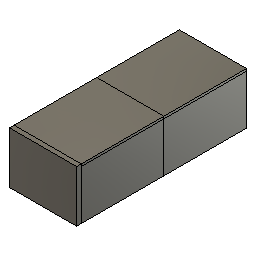
return_to_box_split (Autodesk Fusion 360 design; units mm, degrees)
Autodesk Fusion 360 part; units mm, degrees
sketch "Sketch1" plane through (0, 0, 0) normal (0, 0, 1) x (1, 0, 0)
  line L0 (0, 0) -> (117, 0)
  line L1 (117, 0) -> (117, 86)
  line L2 (117, 86) -> (0, 86)
  line L3 (0, 86) -> (0, 0)
  dimension "d1" = 86
  dimension "d2" = 117
  constraint horizontal L0
  constraint vertical L1
  constraint horizontal L2
  constraint vertical L3
  constraint coincident L0.start L3.end
  measures "d1" distance of L0.end L1.end
  measures "d2" distance of L0.start L0.end
extrude "Extrude1" add sketch "Sketch1" along normal blind 5 makes body 1
sketch "Sketch2" plane through (0, 0, 5) normal (0, 0, 1) x (1, 0, 0)
  line L0 (0, 86) -> (0, 0)
  line L1 (0, 0) -> (117, 0)
  line L2 (117, 0) -> (117, 86)
  line L3 (117, 86) -> (0, 86)
  line L4 (5, 86) -> (5, 5)
  line L5 (5, 5) -> (112, 5)
  line L6 (112, 5) -> (112, 86)
  dimension "d9" = 5
  dimension "d12" = 5
  dimension "d13" = 5
  constraint coincident L3 L4.start
  constraint perpendicular L3 L4
  constraint perpendicular L4 L5
  constraint coincident L3 L6.end
  constraint perpendicular L3 L6
  measures "d9" distance of L1 L5
  measures "d12" distance of L0 L4
  measures "d13" distance of L2 L6
extrude "Extrude2" add sketch "Sketch2" along normal blind 283 contours L0 L1 L2 L3 L4 L5 L6 bodies 1
copy_body "Body->Comp2" bodies 1 removing the originals makes body 2 in component "Shell"
ref_plane "WorkPlane1" through (0, 86, 0) normal (0, 1, 0) x (0, 0, 1) in component "Lid"
sketch "Sketch1 (2)" plane through (0, 86, 0) normal (0, 1, 0) x (1, 0, 0) in component "Lid"
  line L0 (0, 0) -> (117, 0)
  line L1 (117, 0) -> (117, -288)
  line L2 (117, -288) -> (0, -288)
  line L3 (0, -288) -> (0, 0)
  dimension "d125" = 117
  dimension "d126" = 288
  constraint horizontal L0
  constraint vertical L1
  constraint horizontal L2
  constraint vertical L3
  constraint coincident L0.start L3.end
  measures "d125" distance of L1.end L2.end
  measures "d126" distance of L0.end L1.end
extrude "Extrude1'" add sketch "Sketch1 (2)" along normal blind 4 separate body makes body 3 in component "Lid"
sketch "Sketch2 (2)" plane through (0, 86, 0) normal (0, -1, 0) x (1, 0, 0) in component "Lid"
  line L0 (117, 288) -> (0, 288)
  line L1 (0, 288) -> (0, 0)
  line L2 (0, 0) -> (117, 0)
  line L3 (117, 0) -> (117, 288)
  line L4 (5.1, 288) -> (111.9, 288)
  line L5 (111.9, 288) -> (111.9, 5.1)
  line L6 (111.9, 5.1) -> (5.1, 5.1)
  line L7 (5.1, 5.1) -> (5.1, 288)
  dimension "d130" = 5.1
  dimension "d131" = 5.1
  dimension "d132" = 5.1
  constraint horizontal L4
  constraint vertical L5
  constraint horizontal L6
  constraint vertical L7
  constraint collinear L0 L4
  measures "d130" distance of L1 L7
  measures "d131" distance of L3 L5
  measures "d132" distance of L2 L6
extrude "Extrude2'" add sketch "Sketch2 (2)" along normal blind 1 contours L0 L4 L5 L6 L7 bodies 3 in component "Lid"
ref_plane "WorkPlane1" through (0, 0, 288) normal (0, 0, 1) x (1, 0, 0) in component "Door"
sketch "Sketch1 (3)" plane through (0, 0, 288) normal (0, 0, 1) x (1, 0, 0) in component "Door"
  line L0 (0, 0) -> (117, 0)
  line L1 (117, 0) -> (117, 90)
  line L2 (117, 90) -> (0, 90)
  line L3 (0, 90) -> (0, 0)
  dimension "d136" = 117
  dimension "d137" = 90
  constraint horizontal L0
  constraint vertical L1
  constraint horizontal L2
  constraint vertical L3
  constraint coincident L0.start L3.end
  measures "d136" distance of L1.end L2.end
  measures "d137" distance of L0.end L1.end
extrude "Extrude1''" add sketch "Sketch1 (3)" along normal blind 8 separate body makes body 4 in component "Door"
sketch "Sketch2 (3)" plane through (0, 0, 288) normal (0, 0, -1) x (-1, 0, 0) in component "Door"
  line L0 (0, 0) -> (0, 90)
  line L1 (0, 90) -> (-117, 90)
  line L2 (-117, 90) -> (-117, 0)
  line L3 (-117, 0) -> (0, 0)
  line L4 (-106, 83) -> (-11, 83)
  line L5 (-11, 83) -> (-11, 8)
  line L6 (-11, 8) -> (-106, 8)
  line L7 (-106, 8) -> (-106, 83)
  dimension "d140" = 7
  dimension "d141" = 8
  dimension "d142" = 11
  dimension "d143" = 11
  constraint horizontal L4
  constraint vertical L5
  constraint horizontal L6
  constraint vertical L7
  measures "d140" distance of L1 L4
  measures "d141" distance of L3 L6
  measures "d142" distance of L0 L5
  measures "d143" distance of L2 L7
extrude "Extrude2''" add sketch "Sketch2 (3)" along normal blind 5 contours L4 L5 L6 L7 bodies 4 in component "Door"
ref_plane "WorkPlane1" through (0, 0, 6) normal (0, 0, 1) x (1, 0, 0) in component "Drawer"
sketch "Sketch1 (4)" plane through (0, 0, 6) normal (0, 0, 1) x (1, 0, 0) in component "Drawer"
  line L0 (5.5, 84) -> (111.5, 84)
  line L1 (111.5, 84) -> (111.5, 5)
  line L2 (111.5, 5) -> (5.5, 5)
  line L3 (5.5, 5) -> (5.5, 84)
  dimension "d147" = 5
  dimension "d148" = 79
  dimension "d149" = 5.5
  dimension "d150" = 106
  constraint horizontal L0
  constraint vertical L1
  constraint horizontal L2
  constraint vertical L3
  measures "d147" distance of origin L2
  measures "d148" distance of L0.start L2.end
  measures "d149" distance of origin L3
  measures "d150" distance of L0.start L0.end
extrude "Extrude1'''" add sketch "Sketch1 (4)" along normal blind 5 separate body makes body 5 in component "Drawer"
sketch "Sketch2 (4)" plane through (0, 0, 11) normal (0, 0, 1) x (1, 0, 0) in component "Drawer"
  line L0 (5.5, 5) -> (111.5, 5)
  line L1 (111.5, 5) -> (111.5, 84)
  line L2 (111.5, 84) -> (5.5, 84)
  line L3 (5.5, 84) -> (5.5, 5)
  line L4 (10.5, 84) -> (10.5, 8)
  line L5 (10.5, 8) -> (106.5, 8)
  line L6 (106.5, 8) -> (106.5, 84)
  dimension "d153" = 5
  dimension "d154" = 5
  dimension "d155" = 3
  constraint coincident L2 L4.start
  constraint perpendicular L2 L4
  constraint perpendicular L4 L5
  constraint coincident L2 L6.end
  constraint perpendicular L2 L6
  measures "d153" distance of L3 L4
  measures "d154" distance of L1 L6
  measures "d155" distance of L0 L5
extrude "Extrude2'''" add sketch "Sketch2 (4)" along normal blind 277 contours L0 L1 L2 L3 L4 L5 L6 bodies 5 in component "Drawer"
sketch "Sketch3" plane through (111.5, 0, 0) normal (1, 0, 0) x (0, 0, -1) in component "Drawer"
  line L0 (-6, 5) -> (-6, 84)
  line L1 (-6, 84) -> (-288, 84)
  line L2 (-288, 84) -> (-288, 5)
  line L3 (-288, 5) -> (-6, 5)
  line L4 (-258, 84) -> (-258, 49)
  line L5 (-258, 49) -> (-46, 49)
  line L6 (-46, 49) -> (-46, 82)
  line L7 (-46, 82) -> (-6, 82)
  dimension "d158" = 35
  dimension "d159" = 30
  dimension "d160" = 40
  dimension "d351" = 2
  constraint coincident L1 L4.start
  constraint perpendicular L1 L4
  constraint perpendicular L4 L5
  constraint coincident L0 L7.end
  constraint perpendicular L0 L7
  measures "d158" distance of L4.start L4.end
  measures "d159" distance of L2 L4
  measures "d160" distance of L0 L6
  measures "d351" distance of L1 L6.end
extrude "Extrude3" cut sketch "Sketch3" against normal blind 117 contours L0 L1 L4 L5 L6 L7 bodies 5 in component "Drawer"
fillet "Fillet1" radius 20 4 edges at (109, 49, 46) (8, 49, 46) (8, 49, 258) (109, 49, 258) on bodies 5 in component "Drawer"
fillet "Fillet2" radius 15 2 edges at (109, 84, 258) (8, 84, 258) on bodies 5 in component "Drawer"
fillet "Fillet2" radius 15 2 edges at (8, 82, 46) (109, 82, 46) on bodies 5 in component "Drawer"
sketch "Sketch5" plane through (0, 8, 0) normal (0, 1, 0) x (-1, 0, 0)
  line L0 (-106.5, 11) -> (-10.5, 11)
  line L1 (-10.5, 11) -> (-10.5, 288)
  line L2 (-10.5, 288) -> (-106.5, 288)
  line L3 (-106.5, 288) -> (-106.5, 11)
  line L4 (-10.5, 12.5) -> (-106.5, 12.5)
  line L5 (-10.5, 13.25) -> (-106.5, 13.25)
  dimension "d167" = 1.5
  dimension "d168" = 0.75
  constraint coincident L1 L4.start
  constraint coincident L3 L4.end
  constraint perpendicular L3 L4
  constraint coincident L1 L5.start
  constraint coincident L3 L5.end
  constraint perpendicular L3 L5
  measures "d167" distance of L0 L4
  measures "d168" distance of L4 L5
extrude "Extrude4" add sketch "Sketch5" along normal blind 0.4 contours L1 L3 L4 L5 bodies 5 in component "Drawer"
pattern_linear "R-Pattern1" count 100 spacing 2.7096 along (0, 0, 1) of "Extrude4" in component "Drawer"
sketch "Sketch6" plane through (0, 0, 11) normal (0, 0, 1) x (1, 0, 0)
  line L0 (106.5, 8) -> (106.5, 82)
  line L1 (10.5, 82) -> (10.5, 8)
  line L2 (10.5, 8) -> (106.5, 8)
  line L3 (40.5, 84) -> (40.5, 44)
  line L4 (40.5, 44) -> (76.5, 44)
  line L5 (76.5, 44) -> (76.5, 84)
  line L6 (106.5, 82) -> (10.5, 82)
  dimension "d175" = 30
  dimension "d176" = 30
  constraint perpendicular L3 L4
  measures "d175" distance of L1 L3
  measures "d176" distance of L0 L5
extrude "Extrude5" cut sketch "Sketch6" against normal blind 5 contours L3 L4 L5 L6 bodies 5 in component "Drawer"
fillet "Fillet3" radius 15 2 edges at (40.5, 82, 8.5) (76.5, 82, 8.5) on bodies 5 in component "Drawer"
fillet "Fillet4" radius 25.5 2 edges at (40.5, 44, 8.5) (76.5, 44, 8.5) on bodies 5 in component "Drawer"
sketch "Sketch7" plane through (0, 86, 0) normal (0, -1, 0) x (1, 0, 0)
  line L0 (111.9, 288) -> (111.9, 5.1)
  line L1 (111.9, 5.1) -> (5.1, 5.1)
  line L2 (5.1, 5.1) -> (5.1, 288)
  line L3 (5.1, 288) -> (0, 288)
  line L4 (0, 288) -> (0, 0)
  line L5 (0, 0) -> (117, 0)
  line L6 (117, 0) -> (117, 288)
  line L7 (117, 288) -> (111.9, 288)
  circle A0 centre (114.5, 10) radius 1.25
  circle A1 centre (2.5, 10) radius 1.25
  circle A2 centre (114.5, 278) radius 1.25
  circle A3 centre (2.5, 278) radius 1.25
  circle A4 centre (114.5, 154) radius 1.25
  circle A5 centre (114.5, 134) radius 1.25
  circle A6 centre (2.5, 154) radius 1.25
  circle A7 centre (2.5, 134) radius 1.25
  dimension "d188" = 2.5
  dimension "d189" = 2.5
  dimension "d190" = 10
  dimension "d191" = 2.5
  dimension "d192" = 10
  dimension "d193" = 2.5
  dimension "d194" = 2.5
  dimension "d195" = 2.5
  dimension "d196" = 10
  dimension "d197" = 2.5
  dimension "d198" = 10
  dimension "d199" = 2.5
  dimension "d200" = 134
  dimension "d201" = 134
  dimension "d202" = 2.5
  dimension "d203" = 2.5
  dimension "d204" = 2.5
  dimension "d205" = 2.5
  dimension "d206" = 134
  dimension "d207" = 134
  dimension "d208" = 2.5
  dimension "d209" = 2.5
  dimension "d210" = 2.5
  dimension "d211" = 2.5
  measures "d188" diameter of A0
  measures "d189" distance of L6 A0.centre
  measures "d190" distance of L5 A0.centre
  measures "d191" diameter of A1
  measures "d192" distance of L5 A1.centre
  measures "d193" distance of L4 A1.centre
  measures "d194" diameter of A2
  measures "d195" distance of L6 A2.centre
  measures "d196" distance of L7 A2.centre
  measures "d197" diameter of A3
  measures "d198" distance of L3 A3.centre
  measures "d199" distance of L4 A3.centre
  measures "d200" distance of L7 A4.centre
  measures "d201" distance of L5 A5.centre
  measures "d202" diameter of A4
  measures "d203" diameter of A5
  measures "d204" distance of L6 A5.centre
  measures "d205" distance of L6 A4.centre
  measures "d206" distance of L3 A6.centre
  measures "d207" distance of L5 A7.centre
  measures "d208" diameter of A7
  measures "d209" diameter of A6
  measures "d210" distance of L4 A7.centre
  measures "d211" distance of L4 A6.centre
extrude "Extrude3'" add sketch "Sketch7" along normal blind 3 contours A0 | A1 | A2 | A3 | A4 | A5 | A6 | A7 bodies 3 in component "Lid"
fillet "Fillet1'" radius 1 8 edges at (113.3346, 83, 277.548) (1.3346, 83, 277.548) (1.3346, 83, 153.548) (1.3346, 83, 133.548) (1.3346, 83, 9.548) (113.3346, 83, 9.548) (113.3346, 83, 133.548) (113.3346, 83, 153.548) on bodies 3 in component "Lid"
sketch "Sketch8" plane through (0, 86, 0) normal (0, 1, 0) x (-1, 0, 0)
  line L0 (-117, 0) -> (0, 0)
  line L1 (0, 0) -> (0, 288)
  line L2 (0, 288) -> (-5, 288)
  line L3 (-5, 288) -> (-5, 5)
  line L4 (-5, 5) -> (-112, 5)
  line L5 (-112, 5) -> (-112, 288)
  line L6 (-112, 288) -> (-117, 288)
  line L7 (-117, 288) -> (-117, 0)
  circle A0 centre (-2.5, 10) radius 1.3
  circle A1 centre (-114.5, 10) radius 1.3
  circle A2 centre (-114.5, 278) radius 1.3
  circle A3 centre (-2.5, 278) radius 1.3
  circle A4 centre (-2.5, 134) radius 1.3
  circle A5 centre (-2.5, 154) radius 1.3
  circle A6 centre (-114.5, 134) radius 1.3
  circle A7 centre (-114.5, 154) radius 1.3
  dimension "d216" = 10
  dimension "d217" = 134
  dimension "d219" = 134
  dimension "d220" = 10
  dimension "d221" = 10
  dimension "d222" = 134
  dimension "d223" = 10
  dimension "d224" = 134
  dimension "d225" = 2.6
  dimension "d226" = 2.6
  dimension "d227" = 2.6
  dimension "d228" = 2.6
  dimension "d229" = 2.6
  dimension "d230" = 2.6
  dimension "d231" = 2.6
  dimension "d232" = 2.6
  dimension "d233" = 2.5
  dimension "d234" = 2.5
  dimension "d235" = 2.5
  dimension "d236" = 2.5
  dimension "d237" = 2.5
  dimension "d238" = 2.5
  dimension "d239" = 2.5
  dimension "d240" = 2.5
  measures "d216" distance of L6 A2.centre
  measures "d217" distance of L6 A7.centre
  measures "d219" distance of L2 A5.centre
  measures "d220" distance of L2 A3.centre
  measures "d221" distance of L0 A0.centre
  measures "d222" distance of L0 A4.centre
  measures "d223" distance of L0 A1.centre
  measures "d224" distance of L0 A6.centre
  measures "d225" diameter of A0
  measures "d226" diameter of A1
  measures "d227" diameter of A6
  measures "d228" diameter of A7
  measures "d229" diameter of A4
  measures "d230" diameter of A5
  measures "d231" diameter of A3
  measures "d232" diameter of A2
  measures "d233" distance of L7 A2.centre
  measures "d234" distance of L7 A7.centre
  measures "d235" distance of L7 A6.centre
  measures "d236" distance of L7 A1.centre
  measures "d237" distance of L1 A0.centre
  measures "d238" distance of L1 A4.centre
  measures "d239" distance of L1 A5.centre
  measures "d240" distance of L1 A3.centre
extrude "Extrude1''''" cut sketch "Sketch8" against normal blind 3.1 contours A0 | A1 | A2 | A3 | A4 | A5 | A6 | A7 bodies 2 in component "Shell"
sketch "Sketch9" plane through (0, 0, 288) normal (0, 0, 1) x (1, 0, 0)
  line L0 (10.5, 84) -> (5.5, 84)
  line L1 (5.5, 84) -> (5.5, 5)
  line L2 (5.5, 5) -> (111.5, 5)
  line L3 (111.5, 5) -> (111.5, 84)
  line L4 (111.5, 84) -> (106.5, 84)
  line L5 (106.5, 84) -> (106.5, 8)
  line L6 (106.5, 8) -> (10.5, 8)
  line L7 (10.5, 8) -> (10.5, 84)
  circle A0 centre (8, 74) radius 1.3
  circle A1 centre (8, 20) radius 1.3
  circle A2 centre (109, 69) radius 1.3
  circle A3 centre (109, 20) radius 1.3
  dimension "d243" = 2.6
  dimension "d244" = 2.6
  dimension "d245" = 2.6
  dimension "d246" = 2.6
  dimension "d247" = 2.5
  dimension "d248" = 2.5
  dimension "d249" = 2.5
  dimension "d250" = 2.5
  dimension "d251" = 10
  dimension "d252" = 15
  dimension "d253" = 15
  dimension "d254" = 15
  measures "d243" diameter of A0
  measures "d244" diameter of A1
  measures "d245" diameter of A2
  measures "d246" diameter of A3
  measures "d247" distance of L3 A3.centre
  measures "d248" distance of L3 A2.centre
  measures "d249" distance of L1 A0.centre
  measures "d250" distance of L1 A1.centre
  measures "d251" distance of L0 A0.centre
  measures "d252" distance of L2 A1.centre
  measures "d253" distance of L4 A2.centre
  measures "d254" distance of L2 A3.centre
extrude "Extrude6" cut sketch "Sketch9" against normal blind 3.1 contours A0 | A1 | A2 | A3 bodies 5 in component "Drawer"
sketch "Sketch10" plane through (0, 0, 288) normal (0, 0, -1) x (-1, 0, 0)
  line L0 (-106, 8) -> (-106, 83)
  line L1 (-106, 83) -> (-11, 83)
  line L2 (-11, 83) -> (-11, 8)
  line L3 (-11, 8) -> (-106, 8)
  line L4 (0, 0) -> (0, 90)
  line L5 (0, 90) -> (-117, 90)
  line L6 (-117, 90) -> (-117, 0)
  line L7 (-117, 0) -> (0, 0)
  circle A0 centre (-109, 69) radius 1.25
  circle A1 centre (-8, 74) radius 1.25
  circle A2 centre (-8, 20) radius 1.25
  circle A3 centre (-109, 20) radius 1.25
  dimension "d257" = 8
  dimension "d258" = 21
  dimension "d259" = 2.5
  dimension "d260" = 16
  dimension "d261" = 20
  dimension "d262" = 20
  dimension "d263" = 8
  dimension "d264" = 2.5
  dimension "d265" = 8
  dimension "d266" = 2.5
  dimension "d268" = 8
  dimension "d269" = 2.5
  measures "d257" distance of L6 A0.centre
  measures "d258" distance of L5 A0.centre
  measures "d259" diameter of A0
  measures "d260" distance of L5 A1.centre
  measures "d261" distance of L7 A2.centre
  measures "d262" distance of L7 A3.centre
  measures "d263" distance of L6 A3.centre
  measures "d264" diameter of A3
  measures "d265" distance of L4 A2.centre
  measures "d266" diameter of A2
  measures "d268" distance of L4 A1.centre
  measures "d269" diameter of A1
extrude "Extrude3''" add sketch "Sketch10" along normal blind 3 contours A0 | A1 | A2 | A3 bodies 4 in component "Door"
fillet "Fillet1''" radius 1 4 edges at (110.1654, 68.548, 285) (9.1654, 73.548, 285) (9.1654, 19.548, 285) (110.1654, 19.548, 285) on bodies 4 in component "Door"
ref_plane "WorkPlane1" through (0, 0, 144) normal (0, 0, 1) x (1, 0, 0)
split "Split1" by plane through (0, 0, 144) normal (0, 0, 1) bodies 2 makes body 6 at (39, 0, 192) in component "Shell"
split "Split1'" by plane through (0, 0, 144) normal (0, 0, 1) bodies 3 makes body 7 at (39, 90, 192) in component "Lid"
split "Split1''" by plane through (0, 0, 144) normal (0, 0, 1) bodies 5 makes body 8 at (76.1667, 5, 240) in component "Drawer"
copy_body "Body->Comp1" bodies 3 removing the originals makes body 9 in component "Lid Rear"
copy_body "Body->Comp2'" bodies 7 removing the originals makes body 10 in component "Lid Front"
copy_body "Body->Comp1'" bodies 5 removing the originals makes body 11 in component "Drawer Rear"
copy_body "Body->Comp2''" bodies 8 removing the originals makes body 12 in component "Drawer Front"
copy_body "Body->Comp1''" bodies 2 removing the originals makes body 13 in component "Shell Rear"
copy_body "Body->Comp2'''" bodies 6 removing the originals makes body 14 in component "Shell Front"
sketch "Sketch11" plane through (0, 0, 144) normal (0, 0, 1) x (1, 0, 0)
  line L0 (111.5, 5) -> (111.5, 49)
  line L1 (111.5, 49) -> (106.5, 49)
  line L2 (106.5, 49) -> (106.5, 8)
  line L3 (106.5, 8) -> (10.5, 8)
  line L4 (10.5, 8) -> (10.5, 49)
  line L5 (10.5, 49) -> (5.5, 49)
  line L6 (5.5, 49) -> (5.5, 5)
  line L7 (5.5, 5) -> (111.5, 5)
  circle A0 centre (8, 39) radius 1.3
  circle A1 centre (8, 15) radius 1.3
  circle A2 centre (109, 39) radius 1.3
  circle A3 centre (109, 15) radius 1.3
  dimension "d275" = 2.6
  dimension "d276" = 2.6
  dimension "d277" = 2.6
  dimension "d278" = 2.6
  dimension "d279" = 2.5
  dimension "d280" = 2.5
  dimension "d281" = 2.5
  dimension "d282" = 2.5
  dimension "d283" = 10
  dimension "d284" = 10
  dimension "d285" = 10
  dimension "d286" = 10
  measures "d275" diameter of A0
  measures "d276" diameter of A1
  measures "d277" diameter of A2
  measures "d278" diameter of A3
  measures "d279" distance of L0 A2.centre
  measures "d280" distance of L0 A3.centre
  measures "d281" distance of L6 A0.centre
  measures "d282" distance of L6 A1.centre
  measures "d283" distance of L5 A0.centre
  measures "d284" distance of L7 A1.centre
  measures "d285" distance of L1 A2.centre
  measures "d286" distance of L7 A3.centre
extrude "Extrude1'''''" cut sketch "Sketch11" against normal blind 3.1 contours A0 | A1 | A2 | A3 bodies 11 in component "Drawer Rear"
sketch "Sketch12" plane through (0, 0, 144) normal (0, 0, -1) x (-1, 0, 0)
  line L0 (-111.5, 49) -> (-111.5, 5)
  line L1 (-111.5, 5) -> (-5.5, 5)
  line L2 (-5.5, 5) -> (-5.5, 49)
  line L3 (-5.5, 49) -> (-10.5, 49)
  line L4 (-10.5, 49) -> (-10.5, 8)
  line L5 (-10.5, 8) -> (-106.5, 8)
  line L6 (-106.5, 8) -> (-106.5, 49)
  line L7 (-106.5, 49) -> (-111.5, 49)
  circle A0 centre (-109, 39) radius 1.3
  circle A1 centre (-109, 15) radius 1.3
  circle A2 centre (-8, 39) radius 1.3
  circle A3 centre (-8, 15) radius 1.3
  dimension "d289" = 2.6
  dimension "d290" = 2.6
  dimension "d291" = 2.6
  dimension "d292" = 2.6
  dimension "d293" = 2.5
  dimension "d294" = 2.5
  dimension "d295" = 2.5
  dimension "d296" = 2.5
  dimension "d297" = 10
  dimension "d298" = 10
  dimension "d299" = 10
  dimension "d300" = 10
  measures "d289" diameter of A0
  measures "d290" diameter of A1
  measures "d291" diameter of A2
  measures "d292" diameter of A3
  measures "d293" distance of L2 A2.centre
  measures "d294" distance of L2 A3.centre
  measures "d295" distance of L0 A0.centre
  measures "d296" distance of L0 A1.centre
  measures "d297" distance of L7 A0.centre
  measures "d298" distance of L1 A1.centre
  measures "d299" distance of L1 A3.centre
  measures "d300" distance of L3 A2.centre
extrude "Extrude1''''''" cut sketch "Sketch12" against normal blind 3.1 contours A0 | A1 | A2 | A3 bodies 12 in component "Drawer Front"
sketch "Sketch13" plane through (0, 0, 144) normal (0, 0, 1) x (1, 0, 0)
  line L0 (5, 5) -> (5, 86)
  line L1 (5, 86) -> (0, 86)
  line L2 (0, 86) -> (0, 0)
  line L3 (0, 0) -> (117, 0)
  line L4 (117, 0) -> (117, 86)
  line L5 (117, 86) -> (112, 86)
  line L6 (112, 86) -> (112, 5)
  line L7 (112, 5) -> (5, 5)
  circle A0 centre (2.5, 76) radius 1.3
  circle A1 centre (2.5, 10) radius 1.3
  circle A2 centre (114.5, 76) radius 1.3
  circle A3 centre (114.5, 10) radius 1.3
  circle A4 centre (29.25, 2.5) radius 1.3
  circle A5 centre (87.75, 2.5) radius 1.3
  dimension "d303" = 2.6
  dimension "d304" = 2.6
  dimension "d305" = 2.6
  dimension "d306" = 2.6
  dimension "d307" = 2.5
  dimension "d308" = 2.5
  dimension "d309" = 2.5
  dimension "d310" = 2.5
  dimension "d311" = 10
  dimension "d312" = 10
  dimension "d313" = 10
  dimension "d314" = 10
  dimension "d315" = 2.6
  dimension "d316" = 2.6
  dimension "d317" = 2.5
  dimension "d318" = 2.5
  dimension "d319" = 29.25
  dimension "d320" = 29.25
  measures "d303" diameter of A0
  measures "d304" diameter of A1
  measures "d305" diameter of A2
  measures "d306" diameter of A3
  measures "d307" distance of L2 A0.centre
  measures "d308" distance of L2 A1.centre
  measures "d309" distance of L4 A2.centre
  measures "d310" distance of L4 A3.centre
  measures "d311" distance of L1 A0.centre
  measures "d312" distance of L5 A2.centre
  measures "d313" distance of L3 A3.centre
  measures "d314" distance of L3 A1.centre
  measures "d315" diameter of A4
  measures "d316" diameter of A5
  measures "d317" distance of L3 A4.centre
  measures "d318" distance of L3 A5.centre
  measures "d319" distance of L2 A4.centre
  measures "d320" distance of L4 A5.centre
extrude "Extrude1'''''''" [suppressed] in component "Shell Rear"
sketch "Sketch14" plane through (0, 0, 144) normal (0, 0, -1) x (-1, 0, 0)
  line L0 (-5, 86) -> (-5, 5)
  line L1 (-5, 5) -> (-112, 5)
  line L2 (-112, 5) -> (-112, 86)
  line L3 (-112, 86) -> (-117, 86)
  line L4 (-117, 86) -> (-117, 0)
  line L5 (-117, 0) -> (0, 0)
  line L6 (0, 0) -> (0, 86)
  line L7 (0, 86) -> (-5, 86)
  circle A0 centre (-114.5, 76) radius 1.3
  circle A1 centre (-114.5, 10) radius 1.3
  circle A2 centre (-87.75, 2.5) radius 1.3
  circle A3 centre (-29.25, 2.5) radius 1.3
  circle A4 centre (-2.5, 10) radius 1.3
  circle A5 centre (-2.5, 76) radius 1.3
  dimension "d323" = 2.6
  dimension "d324" = 2.6
  dimension "d325" = 2.6
  dimension "d326" = 2.6
  dimension "d327" = 2.6
  dimension "d328" = 2.6
  dimension "d329" = 2.5
  dimension "d330" = 2.5
  dimension "d331" = 2.5
  dimension "d332" = 2.5
  dimension "d333" = 2.5
  dimension "d334" = 2.5
  dimension "d335" = 10
  dimension "d336" = 10
  dimension "d337" = 10
  dimension "d338" = 10
  dimension "d339" = 29.25
  dimension "d340" = 29.25
  measures "d323" diameter of A0
  measures "d324" diameter of A1
  measures "d325" diameter of A2
  measures "d326" diameter of A3
  measures "d327" diameter of A4
  measures "d328" diameter of A5
  measures "d329" distance of L4 A0.centre
  measures "d330" distance of L4 A1.centre
  measures "d331" distance of L6 A4.centre
  measures "d332" distance of L6 A5.centre
  measures "d333" distance of L5 A3.centre
  measures "d334" distance of L5 A2.centre
  measures "d335" distance of L3 A0.centre
  measures "d336" distance of L7 A5.centre
  measures "d337" distance of L5 A4.centre
  measures "d338" distance of L5 A1.centre
  measures "d339" distance of L4 A2.centre
  measures "d340" distance of L6 A3.centre
extrude "Extrude1''''''''" [suppressed] in component "Shell Front"
sketch "Sketch1 (5)" plane through (0, 0, 0) normal (0, 1, 0) x (1, 0, 0) in component "Pin"
  circle A0 centre (0, 0) radius 1.25
  dimension "d343" = 2.5
  constraint coincident A0.centre origin
  measures "d343" diameter of A0
extrude "Extrude1'''''''''" [suppressed] in component "Pin"
move_body "Move1" [suppressed] in component "Pin"
component "Lid" placed x (1, 0, 0) y (0, 1, 0) z (0, 0, 1) at (0, 0, 0)
component "Door" placed x (1, 0, 0) y (0, 1, 0) z (0, 0, 1) at (0, 0, 0)
component "Shell" placed x (1, 0, 0) y (0, 1, 0) z (0, 0, 1) at (0, 0, 0)
component "Drawer" placed x (1, 0, 0) y (0, 1, 0) z (0, 0, 1) at (0, 0, 0)
component "Shell Rear" placed x (1, 0, 0) y (0, 1, 0) z (0, 0, 1) at (0, 0, 0) in component "Shell"
component "Shell Front" placed x (1, 0, 0) y (0, 1, 0) z (0, 0, 1) at (0, 0, 0) in component "Shell"
component "Lid Rear" placed x (1, 0, 0) y (0, 1, 0) z (0, 0, 1) at (0, 0, 0) in component "Lid"
component "Lid Front" placed x (1, 0, 0) y (0, 1, 0) z (0, 0, 1) at (0, 0, 0) in component "Lid"
component "Drawer Rear" placed x (1, 0, 0) y (0, 1, 0) z (0, 0, 1) at (0, 0, 0) in component "Drawer"
component "Drawer Front" placed x (1, 0, 0) y (0, 1, 0) z (0, 0, 1) at (0, 0, 0) in component "Drawer"
equation "d1 = shell_outer_height - lid_thickness"
equation "d2 = shell_outer_width"
equation "d3 = shell_rear_wall_thickness"
equation "shell_rear_wall_thickness = 5 mm"
equation "shell_outer_width = 117 mm"
equation "shell_outer_height = 90 mm"
equation "lid_thickness = 4 mm"
equation "d9 = shell_base_thickness"
equation "shell_base_thickness = 5 mm"
equation "shell_side_wall_thickness = 5 mm"
equation "d12 = shell_side_wall_thickness"
equation "d13 = shell_side_wall_thickness"
equation "door_thickness = 8 mm"
equation "shell_outer_length = 296 mm"
equation "d16 = shell_outer_length - shell_rear_wall_thickness - door_thickness"
equation "drawer_tolerance_side = 0.5 mm"
equation "drawer_tolerance_top = 1 mm"
equation "lid_underhang = 1 mm"
equation "drawer_rear_wall_thickness = 5 mm"
equation "drawer_base_thickness = 3 mm"
equation "drawer_side_wall_thickness = 5 mm"
equation "drawer_tolerance_rear = 1 mm"
equation "door_plug_thickness = 5 mm"
equation "drawer_cut_start = 20 mm"
equation "drawer_cut_depth = 35 mm"
equation "lid_tolerance = 0.1 mm"
equation "drawer_ridge_width = 0.75 mm"
equation "drawer_ridge_height = 0.4 mm"
equation "drawer_ridge_spacing = 1.5 mm"
equation "drawer_ridge_count = 100"
equation "door_side_tolerance = 0.5 mm"
equation "door_top_tolerance = 1 mm"
equation "d124 = shell_outer_height - lid_thickness"
equation "d125 = shell_outer_width"
equation "d126 = shell_outer_length - door_thickness"
equation "d127 = lid_thickness"
equation "d130 = shell_side_wall_thickness + lid_tolerance"
equation "d131 = shell_side_wall_thickness + lid_tolerance"
equation "d132 = shell_rear_wall_thickness + lid_tolerance"
equation "d133 = lid_underhang"
equation "d135 = shell_outer_length - door_thickness"
equation "d136 = shell_outer_width"
equation "d137 = shell_outer_height"
equation "d138 = door_thickness"
equation "d140 = lid_thickness + door_top_tolerance + lid_underhang + drawer_tolerance_top"
equation "d141 = shell_base_thickness + drawer_base_thickness"
equation "d142 = shell_side_wall_thickness + drawer_side_wall_thickness + drawer_tolerance_side + door_side_tolerance"
equation "d143 = shell_side_wall_thickness + drawer_side_wall_thickness + drawer_tolerance_side + door_side_tolerance"
equation "d144 = door_plug_thickness"
equation "d146 = shell_rear_wall_thickness + drawer_tolerance_rear"
equation "d147 = shell_base_thickness"
equation "d148 = shell_outer_height - shell_base_thickness - lid_thickness - lid_underhang - drawer_tolerance_top"
equation "d149 = shell_side_wall_thickness + drawer_tolerance_side"
equation "d150 = shell_outer_width - ( 2 * shell_side_wall_thickness ) - ( 2 * drawer_tolerance_side )"
equation "d151 = drawer_rear_wall_thickness"
equation "d153 = drawer_side_wall_thickness"
equation "d154 = drawer_side_wall_thickness"
equation "d155 = drawer_base_thickness"
equation "d156 = shell_outer_length - shell_rear_wall_thickness - drawer_tolerance_rear - drawer_rear_wall_thickness - door_thickness"
equation "d161 = -shell_outer_width"
equation "d167 = drawer_ridge_spacing"
equation "d168 = drawer_ridge_width"
equation "d169 = drawer_ridge_height"
equation "d171 = drawer_ridge_count"
equation "d173 = -( shell_outer_length - shell_rear_wall_thickness - drawer_tolerance_rear - drawer_rear_wall_thickness - door_plug_thickness - door_thickness - drawer_ridge_spacing - drawer_ridge_spacing - drawer_ridge_width )"
equation "d178 = -shell_rear_wall_thickness"
equation "pin_diameter = 2.5 mm"
equation "pin_depth = 3 mm"
equation "pin_depth_tolerance = 0.1 mm"
equation "pin_diameter_tolerance = 0.1 mm"
equation "d188 = pin_diameter"
equation "d189 = shell_side_wall_thickness / 2"
equation "d191 = pin_diameter"
equation "d193 = shell_side_wall_thickness / 2"
equation "d194 = pin_diameter"
equation "d195 = shell_side_wall_thickness / 2"
equation "d197 = pin_diameter"
equation "d199 = shell_side_wall_thickness / 2"
equation "d200 = ( shell_outer_length - door_thickness ) / 2 - 10 mm"
equation "d201 = ( shell_outer_length - door_thickness ) / 2 - 10 mm"
equation "d202 = pin_diameter"
equation "d203 = pin_diameter"
equation "d204 = shell_side_wall_thickness / 2"
equation "d205 = shell_side_wall_thickness / 2"
equation "d206 = ( shell_outer_length - door_thickness ) / 2 - 10 mm"
equation "d207 = ( shell_outer_length - door_thickness ) / 2 - 10 mm"
equation "d208 = pin_diameter"
equation "d209 = pin_diameter"
equation "d210 = shell_side_wall_thickness / 2"
equation "d211 = shell_side_wall_thickness / 2"
equation "d212 = pin_depth"
equation "d217 = ( shell_outer_length - door_thickness ) / 2 - 10 mm"
equation "d219 = ( shell_outer_length - door_thickness ) / 2 - 10 mm"
equation "d222 = ( shell_outer_length - door_thickness ) / 2 - 10 mm"
equation "d224 = ( shell_outer_length - door_thickness ) / 2 - 10 mm"
equation "d225 = pin_diameter + pin_diameter_tolerance"
equation "d226 = pin_diameter + pin_diameter_tolerance"
equation "d227 = pin_diameter + pin_diameter_tolerance"
equation "d228 = pin_diameter + pin_diameter_tolerance"
equation "d229 = pin_diameter + pin_diameter_tolerance"
equation "d230 = pin_diameter + pin_diameter_tolerance"
equation "d231 = pin_diameter + pin_diameter_tolerance"
equation "d232 = pin_diameter + pin_diameter_tolerance"
equation "d233 = shell_side_wall_thickness / 2"
equation "d234 = shell_side_wall_thickness / 2"
equation "d235 = shell_side_wall_thickness / 2"
equation "d236 = shell_side_wall_thickness / 2"
equation "d237 = shell_side_wall_thickness / 2"
equation "d238 = shell_side_wall_thickness / 2"
equation "d239 = shell_side_wall_thickness / 2"
equation "d240 = shell_side_wall_thickness / 2"
equation "d241 = -pin_depth - pin_depth_tolerance"
equation "d243 = pin_diameter + pin_diameter_tolerance"
equation "d244 = pin_diameter + pin_diameter_tolerance"
equation "d245 = pin_diameter + pin_diameter_tolerance"
equation "d246 = pin_diameter + pin_diameter_tolerance"
equation "d247 = drawer_side_wall_thickness / 2"
equation "d248 = drawer_side_wall_thickness / 2"
equation "d249 = drawer_side_wall_thickness / 2"
equation "d250 = drawer_side_wall_thickness / 2"
equation "d255 = -pin_depth - pin_depth_tolerance"
equation "d257 = shell_side_wall_thickness + drawer_tolerance_side + drawer_side_wall_thickness / 2"
equation "d258 = lid_thickness + lid_underhang + drawer_tolerance_top + 15 mm"
equation "d259 = pin_diameter"
equation "d260 = lid_thickness + lid_underhang + drawer_tolerance_top + 10 mm"
equation "d261 = shell_base_thickness + 15 mm"
equation "d262 = shell_base_thickness + 15 mm"
equation "d263 = shell_side_wall_thickness + drawer_tolerance_side + drawer_side_wall_thickness / 2"
equation "d264 = pin_diameter"
equation "d265 = shell_side_wall_thickness + drawer_tolerance_side + drawer_side_wall_thickness / 2"
equation "d266 = pin_diameter"
equation "d268 = shell_side_wall_thickness + drawer_tolerance_side + drawer_side_wall_thickness / 2"
equation "d269 = pin_diameter"
equation "d270 = pin_depth"
equation "d274 = ( shell_outer_length - door_thickness ) / 2"
equation "d275 = pin_diameter + pin_diameter_tolerance"
equation "d276 = pin_diameter + pin_diameter_tolerance"
equation "d277 = pin_diameter + pin_diameter_tolerance"
equation "d278 = pin_diameter + pin_diameter_tolerance"
equation "d279 = drawer_side_wall_thickness / 2"
equation "d280 = drawer_side_wall_thickness / 2"
equation "d281 = drawer_side_wall_thickness / 2"
equation "d282 = drawer_side_wall_thickness / 2"
equation "d287 = -pin_depth - pin_depth_tolerance"
equation "d289 = pin_diameter + pin_diameter_tolerance"
equation "d290 = pin_diameter + pin_diameter_tolerance"
equation "d291 = pin_diameter + pin_diameter_tolerance"
equation "d292 = pin_diameter + pin_diameter_tolerance"
equation "d293 = drawer_side_wall_thickness / 2"
equation "d294 = drawer_side_wall_thickness / 2"
equation "d295 = drawer_side_wall_thickness / 2"
equation "d296 = drawer_side_wall_thickness / 2"
equation "d301 = -pin_depth - pin_depth_tolerance"
equation "d303 = pin_diameter + pin_diameter_tolerance"
equation "d304 = pin_diameter + pin_diameter_tolerance"
equation "d305 = pin_diameter + pin_diameter_tolerance"
equation "d306 = pin_diameter + pin_diameter_tolerance"
equation "d307 = shell_side_wall_thickness / 2"
equation "d308 = shell_side_wall_thickness / 2"
equation "d309 = shell_side_wall_thickness / 2"
equation "d310 = shell_side_wall_thickness / 2"
equation "d315 = pin_diameter + pin_diameter_tolerance"
equation "d316 = pin_diameter + pin_diameter_tolerance"
equation "d317 = shell_base_thickness / 2"
equation "d318 = shell_base_thickness / 2"
equation "d319 = shell_outer_width / 4"
equation "d320 = shell_outer_width / 4"
equation "d321 = -pin_depth - pin_depth_tolerance"
equation "d323 = pin_diameter + pin_diameter_tolerance"
equation "d324 = pin_diameter + pin_diameter_tolerance"
equation "d325 = pin_diameter + pin_diameter_tolerance"
equation "d326 = pin_diameter + pin_diameter_tolerance"
equation "d327 = pin_diameter + pin_diameter_tolerance"
equation "d328 = pin_diameter + pin_diameter_tolerance"
equation "d329 = shell_side_wall_thickness / 2"
equation "d330 = shell_side_wall_thickness / 2"
equation "d331 = shell_side_wall_thickness / 2"
equation "d332 = shell_side_wall_thickness / 2"
equation "d333 = shell_base_thickness / 2"
equation "d334 = shell_base_thickness / 2"
equation "d339 = shell_outer_width / 4"
equation "d340 = shell_outer_width / 4"
equation "d341 = -pin_depth - pin_depth_tolerance"
equation "d343 = pin_diameter"
equation "d344 = pin_depth * 2"
equation "drawer_tolerance_extra_top_rear = 2 mm"
equation "d351 = drawer_tolerance_extra_top_rear"
